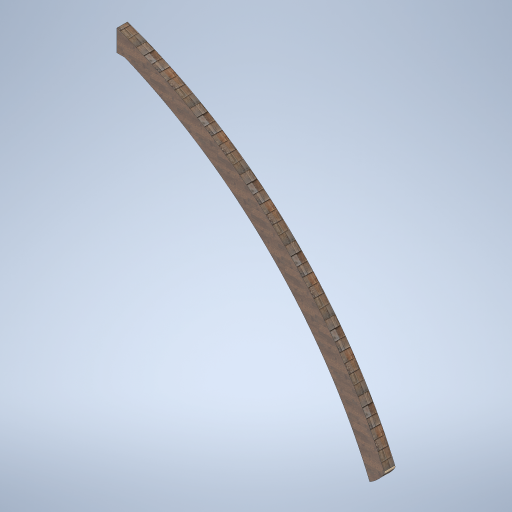
# Autodesk Inventor part: curve_beam
Saved by Autodesk Inventor 2024.2 (Build 282272000, 272)
## iProperties
Created: 2024-05-18
Part Number: curve_beam
Material: Wood Shake
Document SubType Name: Modeling
Designer: LOSTER_1
Density: 0.4 g/cm^3
Appearance: Shake - Handsplit
Author: LOSTER_1
Autodesk Inventor part; units mm, degrees
ref_plane "YZ Plane" through (0, 0, 0) normal (1, 0, 0) x (0, 1, 0)
ref_plane "XZ Plane" through (0, 0, 0) normal (0, 1, 0) x (-1, 0, 0)
ref_plane "XY Plane" through (0, 0, 0) normal (0, 0, 1) x (1, 0, 0)
sketch "Sketch2" plane through (0, 0, 0) normal (0, 0, 1) x (1, 0, 0)
  arc A0 (5000, -4000) -> (0, 700.233) centre (-2826.475, -7316.0653) ccw
  arc A1 (4600, -4000) -> (149.7898, 300.1107) centre (-3126.3122, -7543.1766) ccw
  arc A2 (4720.2587, -4274.9468) -> (4600, -4000) centre (-3126.3122, -7543.1766) ccw
  arc A3 (4720.2587, -4274.9468) -> (5000, -4000) centre (4316.4662, -3584.3299) ccw
  line L0 (149.7898, 300.1107) -> (0, 300.1107)
  line L1 (0, 300.1107) -> (0, 700.233)
  point P0 (0, 0)
  point P1 (4000, -4000)
  dimension "d5" = 8500
  dimension "d7" = 8500
  dimension "d8" = 800
  constraints: 8 point on circle, 4 centre point, 4 end point, 1 horizontal, 1 perpendicular
  measures "d5" radius of A0
  measures "d7" radius of A1
  measures "d8" radius of A3
extrude "Extrusion1" add sketch "Sketch2" along normal blind 100 and the other way blind 100
fillet "Fillet2" radius 50 2 edges at (5000, -4000, 50) (5000, -4000, -50)
body "Solid1"
